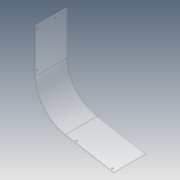
# Autodesk Inventor part: GE-12070-03
Saved by Autodesk Inventor 2012 (Build 160160000, 160)
## iProperties
Created: 2011-09-22
Part Number: GE-12070-03
Document SubType Name: Modeling
Designer: dfoster
Density: 1 g/cm^3
Description: Back
Material: Default
Title: Back
Author: dfoster
Autodesk Inventor part; units mm, degrees
ref_plane "YZ Plane" through (0, 0, 0) normal (1, 0, 0) x (0, 1, 0)
ref_plane "XZ Plane" through (0, 0, 0) normal (0, 1, 0) x (-1, 0, 0)
ref_plane "XY Plane" through (0, 0, 0) normal (0, 0, 1) x (1, 0, 0)
sketch "Sketch1" plane through (0, 0, 0) normal (0, 0, 1) x (1, 0, 0)
  line L0 (-58.6709, 290.177) -> (-55.4959, 290.177) projected
  line L1 (-58.6709, 290.177) -> (-58.6709, 129.0683) projected
  arc A0 (-58.6709, 129.0683) -> (52.835, -3.8192) centre (76.2666, 129.0683) ccw projected
  line L2 (52.835, -3.8192) -> (231.8416, -35.3829) projected
  line L3 (231.8416, -32.1589) -> (231.8416, -35.3829) projected
  line L4 (231.8416, -32.1589) -> (53.3863, -0.6924) projected
  arc A1 (-55.4959, 129.0683) -> (53.3863, -0.6924) centre (76.2666, 129.0683) ccw projected
  line L5 (-55.4959, 129.0683) -> (-55.4959, 290.177) projected
  point P0 (0, 0)
extrude "Extrusion1" add sketch "Sketch1" along normal blind 117.475
hole "Hole1" at (-55.4959, 277.477, 109.5375) direction (-1, 0, 0) diameter 6.731 depth 25.4 tip angle 118
pattern_linear "Rectangular Pattern1" count 2 spacing 133.35 along (0, -1, 0) of "Hole1"
pattern_linear "Rectangular Pattern2" count 2 spacing 68.2625 along (0, 0, -1) of "Hole1"
hole "Hole2" at (219.3346, -29.9536, 109.5375) direction (-0.1736482, -0.9848078, 0) diameter 6.731 depth 25.4 tip angle 118
pattern_linear "Rectangular Pattern4" count 2 spacing 133.35 along (-0.9848078, 0.1736482, 0) of "Hole2"
body "Solid1"
